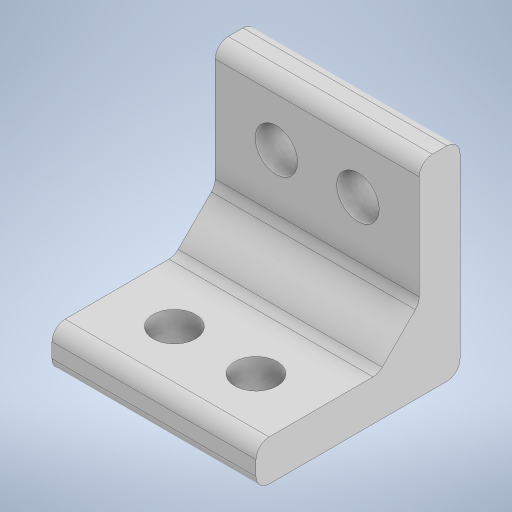
# Autodesk Inventor part: motor_rig_v2
Saved by Autodesk Inventor 2024.2 (Build 282272000, 272)
## iProperties
Created: 2024-02-26
Part Number: motor_rig_v2
Material: Ogólny
Document SubType Name: Modeling
Designer: Konrad
Density: 1 g/cm^3
Appearance: Domyślna
Author: Konrad
Autodesk Inventor part; units mm, degrees
ref_plane "YZ Plane" through (0, 0, 0) normal (1, 0, 0) x (0, 1, 0)
ref_plane "XZ Plane" through (0, 0, 0) normal (0, 1, 0) x (-1, 0, 0)
ref_plane "XY Plane" through (0, 0, 0) normal (0, 0, 1) x (1, 0, 0)
sketch "Szkic1" plane through (0, 0, 0) normal (0, 0, 1) x (1, 0, 0)
  line L0 (0, 0) -> (25, 0)
  line L1 (25, 0) -> (25, 5)
  line L2 (25, 5) -> (0, 5)
  line L3 (0, 5) -> (0, 0)
  line L4 (0, 5) -> (25, 5)
  line L5 (25, 5) -> (25, 25)
  line L6 (25, 25) -> (0, 25)
  line L7 (0, 25) -> (0, 5)
  dimension "d0" = 5
  dimension "d1" = 25
  dimension "d2" = 20
  constraints: 16 end point, 4 parallel, 2 horizontal, 2 perpendicular, 1 point on line
  measures "d0" distance between parallel lines of L0 L2
  measures "d1" distance of L0.start L0.end
  measures "d2" distance of L6.end L2.end
extrude "Wyciągnięcie proste1" add sketch "Szkic1" along normal blind 5 contours L7 L6 L5 L2
extrude "Wyciągnięcie proste2" add sketch "Szkic1" along normal blind 25 contours L3 L2 L1 L0
chamfer "Faza1" distance 5 angle 45 1 edges at (12.5, 5, 5)
sketch "Szkic2" plane through (0, 5, 25) normal (0, 1, 0) x (1, 0, 0)
  line L0 (0, 15) -> (25, 15) projected
  line L1 (0, 15) -> (0, 0) projected
  line L2 (25, 0) -> (0, 0) projected
  line L3 (25, 15) -> (25, 0) projected
  line L4 (25, 0) -> (0, 0) projected
  line L5 (12.5, 0) -> (12.5, 15)
  circle A0 centre (7.5, 7.5) radius 2.6
  circle A1 centre (17.5, 7.5) radius 2.6
  point P0 (0, 25)
  dimension "d10" = 5.2
  dimension "d11" = 10
  dimension "d12" = 7.5
  dimension "d21" = 15
  constraints: 2 centre point, 2 end point, 2 midpoint, 1 equal radius, 1 symmetric about line
  measures "d10" diameter of A0
  measures "d11" distance of A1.centre A0.centre
  measures "d12" distance from line of A0.centre L2
  measures "d21" distance of L0.end L2.start
extrude "Wyciągnięcie proste3" cut sketch "Szkic2" against normal up to surface (5 mm away) contours A0 | A1
sketch "Szkic3" plane through (0, 0, 5) normal (0, 0, 1) x (1, 0, 0)
  line L0 (25, 10) -> (0, 10) projected
  line L1 (25, 10) -> (25, 25) projected
  line L2 (25, 25) -> (0, 25) projected
  line L3 (0, 25) -> (0, 10) projected
  circle A0 centre (17.5, 17.5) radius 2.6
  circle A1 centre (7.5, 17.5) radius 2.6
  line L4 (25, 25) -> (0, 25) projected
  line L5 (12.5, 25) -> (12.5, 10)
  point P0 (0, 0)
  dimension "d15" = 5.2
  dimension "d16" = 10
  dimension "d20" = 7.5
  dimension "d22" = 15
  constraints: 2 centre point, 2 end point, 2 midpoint, 1 equal radius, 1 symmetric about line
  measures "d15" diameter of A0
  measures "d16" distance of A1.centre A0.centre
  measures "d20" distance from line of L2 A1.centre
  measures "d22" distance of L0.start L1.end
extrude "Wyciągnięcie proste4" cut sketch "Szkic3" against normal up to surface (5 mm away) contours A0 | A1
fillet "Zaokrąglenie1" radius 1.6 7 edges at (12.5, 0, 0) (12.5, 0, 25) (12.5, 5, 25) (12.5, 5, 10) (12.5, 10, 5) (12.5, 25, 5) (12.5, 25, 0)
equation "\"d12\" = 0.5 * d21"
equation "\"d20\" = 0.5 * d22"
